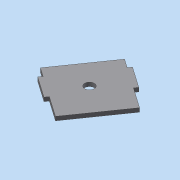
# Autodesk Inventor part: Part7
Saved by Autodesk Inventor 2016 SP1 (Build 200210100, 210)
## iProperties
Created: 2016-03-24
Part Number: Part7
Material: Generic
Document SubType Name: Modeling
Designer: Mohamed A.
Density: 1 g/cm^3
Appearance: Default
Author: Mohamed A.
Autodesk Inventor part; units mm, degrees
ref_plane "YZ Plane" through (0, 0, 0) normal (1, 0, 0) x (0, 1, 0)
ref_plane "XZ Plane" through (0, 0, 0) normal (0, 1, 0) x (-1, 0, 0)
ref_plane "XY Plane" through (0, 0, 0) normal (0, 0, 1) x (1, 0, 0)
sketch "Sketch1" plane through (0, 0, 0) normal (0, 0, 1) x (1, 0, 0)
  circle A0 centre (6.25, 0) radius 10.15 construction
  line L0 (-4.702, -26.1294) -> (1.4519, -30.4166) projected
  line L1 (1.4519, -30.4166) -> (3.1668, -27.9551) projected
  circle A1 centre (6.25, 0) radius 3.75 projected
  line L2 (-17.5496, -17.1789) -> (-11.6763, -21.2706) projected
  line L3 (-11.6763, -21.2706) -> (-9.9615, -18.8091) projected
  line L4 (-9.9615, -18.8091) -> (-7.7051, -20.381) projected
  line L5 (-7.7051, -20.381) -> (-6.5618, -18.74) projected
  line L6 (-6.5618, -18.74) -> (-7.5054, -18.0826) projected
  line L7 (-7.5054, -18.0826) -> (-6.1335, -16.1134) projected
  line L8 (-6.1335, -16.1134) -> (-5.1899, -16.7708) projected
  line L9 (-5.1899, -16.7708) -> (-4.8469, -16.2785) projected
  line L10 (-4.8469, -16.2785) -> (-2.3854, -17.9933) projected
  line L11 (-2.3854, -17.9933) -> (-2.7284, -18.4856) projected
  line L12 (-2.7284, -18.4856) -> (-1.7848, -19.143) projected
  line L13 (-1.7848, -19.143) -> (-3.1567, -21.1123) projected
  line L14 (-3.1567, -21.1123) -> (-4.1003, -20.4549) projected
  line L15 (-4.1003, -20.4549) -> (-5.2435, -22.0959) projected
  line L16 (-5.2435, -22.0959) -> (-2.9871, -23.6679) projected
  line L17 (-2.9871, -23.6679) -> (-4.702, -26.1294) projected
  line L18 (3.1668, -27.9551) -> (12.8078, -34.6717) projected
  line L19 (12.8078, -34.6717) -> (41.0461, 5.8617) projected
  line L20 (41.0461, 5.8617) -> (31.4051, 12.5783) projected
  line L21 (31.4051, 12.5783) -> (33.12, 15.0399) projected
  line L22 (33.12, 15.0399) -> (26.9661, 19.3271) projected
  line L23 (26.9661, 19.3271) -> (25.2512, 16.8655) projected
  line L24 (25.2512, 16.8655) -> (22.9948, 18.4375) projected
  line L25 (22.9948, 18.4375) -> (21.8515, 16.7965) projected
  line L26 (21.8515, 16.7965) -> (22.7951, 16.1391) projected
  line L27 (22.7951, 16.1391) -> (21.4232, 14.1699) projected
  line L28 (21.4232, 14.1699) -> (20.4796, 14.8272) projected
  line L29 (20.4796, 14.8272) -> (20.1367, 14.3349) projected
  line L30 (20.1367, 14.3349) -> (17.6751, 16.0498) projected
  line L31 (17.6751, 16.0498) -> (18.0181, 16.5421) projected
  line L32 (18.0181, 16.5421) -> (17.0745, 17.1995) projected
  line L33 (17.0745, 17.1995) -> (18.4464, 19.1687) projected
  line L34 (18.4464, 19.1687) -> (19.39, 18.5114) projected
  line L35 (19.39, 18.5114) -> (20.5333, 20.1524) projected
  line L36 (20.5333, 20.1524) -> (18.2768, 21.7244) projected
  line L37 (18.2768, 21.7244) -> (19.9917, 24.1859) projected
  line L38 (19.9917, 24.1859) -> (14.1185, 28.2776) projected
  line L39 (14.1185, 28.2776) -> (12.4036, 25.8161) projected
  line L40 (12.4036, 25.8161) -> (2.4819, 32.7281) projected
  line L41 (2.4819, 32.7281) -> (-25.7564, -7.8053) projected
  line L42 (-25.7564, -7.8053) -> (-15.8347, -14.7174) projected
  line L43 (-15.8347, -14.7174) -> (-17.5496, -17.1789) projected
  point P0 (0, 0)
extrude "Extrusion1" add sketch "Sketch1" along normal blind 3
body "Solid1"
